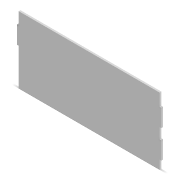
# Autodesk Inventor part: Piso
Saved by Autodesk Inventor 2022 (Build 260153000, 153)
## iProperties
Created: 2022-06-06
Part Number: Piso
Material: Generic
Document SubType Name: Modeling
Designer: ADMIN
Density: 1 g/cm^3
Appearance: Default
Author: ADMIN
Autodesk Inventor part; units mm, degrees
ref_plane "YZ Plane" through (0, 0, 0) normal (1, 0, 0) x (0, 1, 0)
ref_plane "XZ Plane" through (0, 0, 0) normal (0, 1, 0) x (-1, 0, 0)
ref_plane "XY Plane" through (0, 0, 0) normal (0, 0, 1) x (1, 0, 0)
sketch "Sketch1" plane through (0, 0, 0) normal (0, 0, 1) x (1, 0, 0)
  line L0 (505, 160) -> (505, 110) projected
  line L1 (505, 160) -> (500, 160) projected
  line L2 (500, 110) -> (500, 160) projected
  line L3 (505, 110) -> (500, 110) projected
  line L4 (505, 80) -> (505, 30) projected
  line L5 (505, 80) -> (500, 80) projected
  line L6 (500, 30) -> (500, 80) projected
  line L7 (505, 30) -> (500, 30) projected
  line L8 (100, 160) -> (100, 110) projected
  line L9 (100, 160) -> (95, 160) projected
  line L10 (95, 110) -> (95, 160) projected
  line L11 (100, 110) -> (95, 110) projected
  line L12 (100, 80) -> (100, 30) projected
  line L13 (100, 80) -> (95, 80) projected
  line L14 (95, 30) -> (95, 80) projected
  line L15 (100, 30) -> (95, 30) projected
  line L16 (95, 160) -> (100, 160) projected
  line L17 (100, 160) -> (100, 350) projected
  line L18 (100, 350) -> (95, 350) projected
  line L19 (95, 160) -> (95, 350) projected
  line L20 (100, 200) -> (500, 200) projected
  line L21 (500, 200) -> (500, 205) projected
  line L22 (100, 205) -> (500, 205) projected
  line L23 (500, 160) -> (505, 160) projected
  line L24 (505, 160) -> (505, 350) projected
  line L25 (505, 350) -> (500, 350) projected
  line L26 (500, 160) -> (500, 350) projected
  line L27 (505, 0) -> (500, 0) projected
  line L28 (500, 0) -> (500, -5) projected
  line L29 (505, -5) -> (500, -5) projected
  line L30 (505, 0) -> (505, -5) projected
  line L31 (100, 200) -> (500, 200)
  line L32 (500, 200) -> (500, 0)
  line L33 (500, 0) -> (100, 0)
  line L34 (100, 0) -> (100, 200)
  line L35 (500, 195) -> (100, 195)
  line L36 (100, 5) -> (500, 5)
  line L37 (100, 200) -> (100, 205) projected
  point P0 (0, 0)
  point P1 (100, 110)
  point P2 (100, 80)
  point P3 (100, 30)
  point P4 (100, 195)
  point P5 (0, 112.5)
  point P6 (95, 200)
  dimension "d2" = 5
  dimension "d3" = 5
  constraints: 12 end point, 4 point on line, 3 perpendicular, 2 parallel, 1 horizontal
  measures "d2" distance between parallel lines of L33 L36
  measures "d3" distance between parallel lines of L35 L31
extrude "Extrusion1" add sketch "Sketch1" along normal blind 5 contours L0 L3 L2 L1 | L2 L32 L6 L36 L34 L12 L8 L17 L35 L26 | L5 L4 L7 L6 | L8 L11 L10 L9 | L12 L15 L14 L13
body "Solid1"
